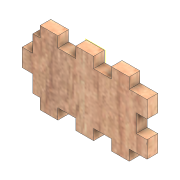
# Autodesk Inventor part: jotstick behuizing zijkant 2
Saved by Autodesk Inventor 2020.3 (Build 243373000, 373)
## iProperties
Created: 2020-12-09
Part Number: jotstick behuizing zijkant 2
Material: Wood (Birch)
Document SubType Name: Sheet Metal
Designer: Svend
Density: 0.55 g/cm^3
Sheet Metal Rule: Default_mm
Appearance: Birch - Natural Polished
Author: Svend
Autodesk Inventor part; units mm, degrees
ref_plane "YZ Plane" through (0, 0, 0) normal (1, 0, 0) x (0, 1, 0)
ref_plane "XZ Plane" through (0, 0, 0) normal (0, 1, 0) x (-1, 0, 0)
ref_plane "XY Plane" through (0, 0, 0) normal (0, 0, 1) x (1, 0, 0)
ref_plane "Work Plane1" through (20, 0, 0) normal (0, 0, 1) x (1, 0, 0)
sketch "Sketch1" plane through (20, 0, 0) normal (0, 0, 1) x (1, 0, 0)
  line L0 (-20, 0) -> (-10, 0)
  line L1 (-10, 0) -> (-10, 6)
  line L2 (-20, 6) -> (-10, 6)
  line L3 (-20, 0) -> (-20, 6)
  line L4 (0, 0) -> (10, 0)
  line L5 (10, 0) -> (10, 6)
  line L6 (0, 6) -> (10, 6)
  line L7 (0, 0) -> (0, 6)
  line L8 (20, 0) -> (30, 0)
  line L9 (30, 0) -> (30, 6)
  line L10 (20, 6) -> (30, 6)
  line L11 (20, 0) -> (20, 6)
  line L12 (-30, 0) -> (-24, 0)
  line L13 (-24, 0) -> (-24, 6)
  line L14 (-30, 6) -> (-24, 6)
  line L15 (-30, 0) -> (-30, 6)
  line L16 (-30, 0) -> (-20, 0)
  line L17 (-10, 0) -> (0, 0)
  line L18 (10, 0) -> (20, 0)
  line L19 (30, 0) -> (40, 0)
  line L20 (40, 0) -> (-24, 0)
  line L21 (-24, 0) -> (-24, -29)
  line L22 (-24, -29) -> (40, -29)
  line L23 (40, -29) -> (40, 0)
  line L24 (-24, -9.5) -> (-30, -9.5)
  line L25 (-30, -9.5) -> (-30, -19.5)
  line L26 (-30, -19.5) -> (-24, -19.5)
  line L27 (-24, -19.5) -> (-24, -9.5)
  line L28 (40, -19.5) -> (34, -19.5)
  line L29 (34, -19.5) -> (34, -9.5)
  line L30 (34, -9.5) -> (40, -9.5)
  line L31 (40, -9.5) -> (40, -19.5)
  line L32 (-24, -14.5) -> (40, -14.5) construction
  line L33 (-20, -29) -> (-10, -29)
  line L34 (-10, -29) -> (-10, -35)
  line L35 (-20, -35) -> (-10, -35)
  line L36 (-20, -29) -> (-20, -35)
  line L37 (0, -29) -> (10, -29)
  line L38 (10, -29) -> (10, -35)
  line L39 (0, -35) -> (10, -35)
  line L40 (0, -29) -> (0, -35)
  line L41 (20, -29) -> (30, -29)
  line L42 (30, -29) -> (30, -35)
  line L43 (20, -35) -> (30, -35)
  line L44 (20, -29) -> (20, -35)
  line L45 (-10, -29) -> (0, -29)
  line L46 (10, -29) -> (20, -29)
  point P0 (-30, -14.5)
  point P1 (34, -14.5)
  dimension "d0" = 29
  dimension "d1" = 6
  dimension "d2" = 10
  measures "d0" distance of L21.end L20.end
  measures "d1" distance of L26.end L25.end
  measures "d2" distance of L25.end L24.end
extrude "Plate1" add sketch "Sketch1" along normal blind 6 contours L3 L2 L1 L0 | L0 L17 L4 L18 L8 L19 L23 L30 L29 L28 L22 L21 L16 | L7 L6 L5 L4 | L21 L26 L25 L24 | L11 L10 L9 L8 | L22 L34 L35 L36 | L22 L38 L39 L40 | L22 L42 L43 L44
equation "\"d3\" = Thickness"
equation "\"BendRadius\" = Thickness"
equation "\"BendReliefWidth\" = Thickness"
equation "\"BendReliefDepth\" = 0.5 * Thickness"
equation "\"CornerReliefSize\" = 4 * Thickness"
equation "\"MinimumRemnant\" = 2 * Thickness"
equation "\"TransitionRadius\" = BendRadius"
equation "\"JacobiRadiusSize\" = BendRadius"
equation "\"GapSize\" = Thickness"
equation "\"Thickness\" = 6"
body "Solid1"
